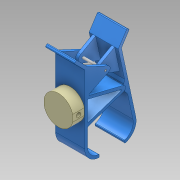
# Autodesk Inventor part: В. шарн. - держатель смартфона
Saved by Autodesk Inventor 2018 (Build 220112000, 112)
## iProperties
Created: 2020-02-22
Part Number: В. шарн. - держатель смартфона
Material: Типовые
Document SubType Name: Modeling
Designer: Leancher
Density: 1 g/cm^3
Appearance: По умолчанию
Author: Leancher
Autodesk Inventor part; units mm, degrees
ref_plane "YZ Plane" through (0, 0, 0) normal (1, 0, 0) x (0, 1, 0)
ref_plane "XZ Plane" through (0, 0, 0) normal (0, 1, 0) x (-1, 0, 0)
ref_plane "XY Plane" through (0, 0, 0) normal (0, 0, 1) x (1, 0, 0)
sketch "Эскиз1" plane through (0, 0, 0) normal (1, 0, 0) x (0, 0, -1)
  line L0 (-5.1487, -13.4444) -> (-9.7487, -13.4444)
  line L1 (-9.7487, -13.4444) -> (-9.7487, -18.4444)
  line L2 (-9.7487, -18.4444) -> (7.2513, -18.4444)
  line L3 (7.2513, -18.4444) -> (7.2513, -13.4444)
  line L4 (7.2513, -13.4444) -> (2.6513, -13.4444)
  line L5 (2.6513, -13.4444) -> (2.6513, -8.4651)
  line L6 (2.6513, -8.4651) -> (7.2513, -8.4651)
  line L7 (7.2513, -8.4651) -> (7.2513, 21.5556)
  line L8 (7.2513, 21.5556) -> (-9.7487, 21.5556)
  line L9 (-9.7487, 21.5556) -> (-9.7487, -8.4237)
  line L10 (-9.7487, -8.4237) -> (-5.1487, -8.4237)
  line L11 (-5.1487, -8.4237) -> (-5.1487, -13.4444)
  circle A0 centre (-1.2487, 17.5556) radius 1
  dimension "d13" = 0.5
  constraints: 24 end point, 1 centre point
sketch "Эскиз2" plane through (0, 0, 0) normal (0, 1, 0) x (-1, 0, 0)
  line L0 (-9.727, -2.3208) -> (-9.727, 2.3208)
  line L1 (9.727, 2.3208) -> (9.727, -2.3208)
  arc A0 (9.727, 2.3208) -> (-9.727, 2.3208) centre (0, 0) ccw
  arc A1 (-9.727, -2.3208) -> (9.727, -2.3208) centre (0, 0) ccw
  constraints: 4 end point, 4 point on circle, 2 centre point, 1 coincident
extrude "Выдавливание2" add sketch "Эскиз2" along normal blind 8
sketch "Эскиз3" plane through (0, 0, 0) normal (1, 0, 0) x (0, 1, 0)
  line L0 (7.8536, 25.1464) -> (1.2825, 31.7175)
  line L1 (1.2825, 32.4246) -> (1.9896, 33.1317)
  line L2 (2.6967, 33.1317) -> (9.9377, 25.8908)
  arc A0 (8, -22) -> (17.4737, -31.9861) centre (18, -22) ccw
  line L3 (8, 24.7929) -> (8, -22)
  line L4 (10, -22) -> (10, -10.3547)
  arc A1 (10, -22) -> (17.5294, -29.9861) centre (18, -22) ccw
  line L5 (18, -30.4853) -> (18, -31.4868)
  line L6 (10.0799, 25.7912) -> (24.3236, 19.1492)
  line L7 (24.3542, 15.5386) -> (11.2398, 9.1501)
  arc A2 (24.3542, 15.5386) -> (24.3236, 19.1492) centre (23.4783, 17.3366) ccw
  line L8 (11.3388, 8.2152) -> (34.5374, 2.4804)
  line L9 (34.7181, -1.3488) -> (10.3348, -9.8828)
  arc A3 (34.7181, -1.3488) -> (34.5374, 2.4804) centre (34.0574, 0.5389) ccw
  line L10 (21.7887, 3.5717) -> (32.825, 0.8435)
  line L11 (21.7887, 3.5717) -> (10.62, 6.3327)
  line L12 (21.7887, -3.7645) -> (10.6564, -7.4318)
  line L13 (21.7887, -3.7645) -> (32.8615, -0.1167)
  line L14 (10, 5.8473) -> (10, -6.957)
  arc A4 (32.8615, -0.1167) -> (32.825, 0.8435) centre (32.7051, 0.3582) ccw
  circle A5 centre (22.3591, 17.3536) radius 0.75
  arc A6 (1.2825, 32.4246) -> (1.2825, 31.7175) centre (1.636, 32.0711) ccw
  arc A7 (2.6967, 33.1317) -> (1.9896, 33.1317) centre (2.3431, 32.7782) ccw
  arc A8 (8, 24.7929) -> (7.8536, 25.1464) centre (7.5, 24.7929) ccw
  arc A9 (9.9377, 25.8908) -> (10.0799, 25.7912) centre (10.2912, 26.2443) ccw
  arc A10 (11.2398, 9.1501) -> (11.3388, 8.2152) centre (11.4588, 8.7006) ccw
  arc A11 (10.62, 6.3327) -> (10, 5.8473) centre (10.5, 5.8473) ccw
  arc A12 (10, -6.957) -> (10.6564, -7.4318) centre (10.5, -6.957) ccw
  arc A13 (10.3348, -9.8828) -> (10, -10.3547) centre (10.5, -10.3547) ccw
  arc A14 (18, -30.4853) -> (17.5294, -29.9861) centre (17.5, -30.4853) ccw
  arc A15 (17.4737, -31.9861) -> (18, -31.4868) centre (17.5, -31.4868) ccw
  point P0 (0, 0)
  point P1 (18, -32)
  point P2 (18, -30)
  dimension "d13" = 0.5
  constraints: 33 point on circle, 30 end point, 26 tangent, 16 centre point, 9 equal radius, 2 point on line, 1 coincident
  measures "d13" radius of A6
extrude "Выдавливание3" add sketch "Эскиз3" along normal mid plane 20 separate body
sketch "Эскиз4" plane through (-10, 10, -6.957) normal (0, 1, 0) x (1, 0, 0)
  line L0 (18, -32.7481) -> (2, -32.7481)
  line L1 (2, -15.1722) -> (2, -32.7481)
  line L2 (18, -15.1722) -> (18, -32.7481)
  line L3 (18, -15.1722) -> (2, -15.1722)
  point P0 (10, -6.957)
  constraints: 8 end point
extrude "Выдавливание4" cut sketch "Эскиз4" along normal blind 20 bodies 1 2
sketch "Эскиз5" plane through (0, 0, 0) normal (1, 0, 0) x (0, 1, 0)
  arc A0 (35.6637, -0.6527) -> (35.1571, 2.2094) centre (34.0574, 0.5389) ccw
  arc A1 (35.4164, -30.3921) -> (41.098, -21.0011) centre (33.2769, -22.6835) ccw
  arc A2 (35.4164, -30.3921) -> (35.0614, -30.979) centre (35.5502, -30.8739) ccw
  line L0 (35.0614, -30.979) -> (35.272, -31.9582)
  arc A3 (35.272, -31.9582) -> (35.8915, -32.3356) centre (35.7608, -31.853) ccw
  arc A4 (35.8915, -32.3356) -> (43.0533, -20.5805) centre (33.2769, -22.6835) ccw
  arc A5 (33.2815, 25.5424) -> (33.2127, 25.166) centre (33.7015, 25.2711) ccw
  line L1 (38.3237, 33.3484) -> (33.2815, 25.5424)
  arc A6 (38.3237, 33.3484) -> (38.175, 34.0397) centre (37.9037, 33.6197) ccw
  line L2 (37.335, 34.5823) -> (38.175, 34.0397)
  arc A7 (37.335, 34.5823) -> (36.6437, 34.4336) centre (37.0637, 34.1623) ccw
  line L3 (31.0396, 25.7578) -> (36.6437, 34.4336)
  line L4 (43.0533, -20.5805) -> (33.2127, 25.166)
  arc A8 (20.8463, 20.0597) -> (21.3193, 14.4329) centre (22.3591, 17.3536) ccw
  line L5 (34.4838, 9.7464) -> (21.3193, 14.4329)
  line L6 (31.0396, 25.7578) -> (20.8463, 20.0597)
  line L7 (35.6973, -1.8871) -> (37.4375, -3.9843)
  line L8 (34.7362, 3.2847) -> (35.3445, 5.7454)
  line L9 (41.098, -21.0011) -> (37.4375, -3.9843)
  line L10 (35.3445, 5.7454) -> (34.4838, 9.7464)
  arc A9 (35.6637, -0.6527) -> (35.6973, -1.8871) centre (36.4668, -1.2485) ccw
  arc A10 (34.7362, 3.2847) -> (35.1571, 2.2094) centre (35.707, 3.0447) ccw
  circle A11 centre (22.3591, 17.3536) radius 0.75
  constraints: 22 end point, 22 point on circle, 12 centre point, 4 tangent, 1 coincident, 1 equal radius
extrude "Выдавливание5" add sketch "Эскиз5" along normal mid plane 20 separate body
sketch "Эскиз6" plane through (-10, 35.3445, 5.7454) normal (0, -0.9776367, -0.2103011) x (1, 0, 0)
  line L0 (10, 1.8161) -> (10, 24.3613) construction
  line L1 (2.5, 20.4701) -> (0, 20.4701)
  line L2 (0, 4.0925) -> (2.5, 4.0925)
  line L3 (2.5, 4.0925) -> (2.5, 20.4701)
  line L4 (17.5, 20.4701) -> (20, 20.4701)
  line L5 (20, 4.0925) -> (17.5, 4.0925)
  line L6 (17.5, 4.0925) -> (17.5, 20.4701)
  line L7 (0, 20.4701) -> (0, 4.0925)
  line L8 (20, 4.0925) -> (20, 20.4701)
  line L9 (0, 19.7881) -> (20, 19.7881) projected
  line L10 (15.5, 20.4701) -> (4.5, 20.4701)
  line L11 (4.5, 20.4701) -> (4.5, 4.0925)
  line L12 (4.5, 4.0925) -> (15.5, 4.0925)
  line L13 (15.5, 4.0925) -> (15.5, 20.4701)
  constraints: 26 end point, 4 symmetric about line
extrude "Выдавливание6" cut sketch "Эскиз6" along normal blind 20 bodies 3
sketch "Эскиз7" plane through (0, 0, 0) normal (1, 0, 0) x (0, 1, 0)
  circle A0 centre (22.3591, 17.3536) radius 0.75 projected
  point P0 (0, 0)
extrude "Выдавливание7" add sketch "Эскиз7" along normal mid plane 20 separate body
sketch "Эскиз8" plane through (9.727, 0, 2.3208) normal (1, 0, 0) x (0, 0, -1)
  circle A0 centre (2.3208, 4) radius 1.5
  constraints: 1 centre point
extrude "Выдавливание8" cut sketch "Эскиз8" against normal blind 20 bodies 1
